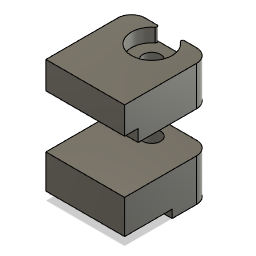
Korthållare_bak v4 (Autodesk Fusion 360 design; units mm, degrees)
Autodesk Fusion 360 part; units mm, degrees
sketch "Sketch1" plane through (0, 0, 0) normal (1, 0, 0) x (0, 0, -1)
  line L0 (0, 0) -> (-5.6, 0)
  line L1 (-5.6, 0) -> (-5.6, 1.2)
  line L2 (-5.6, 1.2) -> (-12.6, 1.2)
  line L3 (-12.6, 1.2) -> (-12.6, 6.2)
  line L4 (-12.6, 6.2) -> (0, 6.2)
  line L5 (0, 6.2) -> (0, 0)
  line L6 (-12.6, 8) -> (-10.6, 8)
  line L7 (-10.6, 8) -> (-10.6, 6.2)
  line L8 (-12.6, 8) -> (-12.6, 12)
  line L9 (-12.6, 12) -> (0, 12)
  line L10 (0, 12) -> (0, 6.2)
  dimension "d1" = 5.6
  dimension "d2" = 1.2
  dimension "d4" = 5
  dimension "d5" = 1.8
  dimension "d6" = 2
  dimension "d7" = 4
  dimension "d24" = 5
  constraint coincident L0.start L5.end
  constraint horizontal L0
  constraint perpendicular L0 L1
  constraint perpendicular L1 L2
  constraint perpendicular L2 L3
  constraint perpendicular L3 L4
  constraint vertical L5
  constraint horizontal L6
  constraint coincident L4 L7.end
  constraint perpendicular L4 L7
  constraint perpendicular L6 L8
  constraint perpendicular L8 L9
  constraint vertical L10
  constraint collinear L3 L8
  measures "d1" distance of L0.start L0.end
  measures "d2" distance of L0.end L1.end
  measures "d4" distance of L2.end L3.end
  measures "d5" distance of L6.end L7.end
  measures "d6" distance of L6.start L6.end
  measures "d7" distance of L6 L9
  measures "d24" distance of L1 L7
extrude "Extrude1" add sketch "Sketch1" along normal blind 11.6 contours L0 L1 L2 L3 L4 L5 makes body 1
extrude "Extrude2" add sketch "Sketch1" along normal blind 11.6 separate body contours L4 L6 L7 L8 L9 L10 makes body 2
sketch "Sketch2" plane through (0, 12, 0) normal (0, 1, 0) x (-1, 0, 0)
  line L0 (0, 0) -> (0, 12.6)
  line L1 (0, 12.6) -> (-11.6, 12.6)
  line L2 (-11.6, 12.6) -> (-11.6, 0)
  line L3 (-11.6, 0) -> (0, 0)
  circle A0 centre (-5.8, 2.8) radius 1.3
  line L4 (-5.8, 2.8) -> (-5.8, 0) construction
  circle A1 centre (-5.8, 2.8) radius 3
  dimension "d12" = 2.6
  dimension "d15" = 2.8
  dimension "d20" = 6
  constraint coincident A0.centre L4.start
  constraint midpoint L3 L4.end
  constraint perpendicular L3 L4
  constraint concentric A0 A1
  measures "d12" diameter of A0
  measures "d15" distance of A0.centre L4.end
  measures "d20" diameter of A1
extrude "Extrude3" cut sketch "Sketch2" against normal blind 18 contours A0 bodies 1 2
extrude "Extrude5" cut sketch "Sketch2" against normal blind 2 contours L3 A1 | L3 A1 bodies 2
sketch "Sketch3" plane through (0, 0, 0) normal (0, -1, 0) x (1, 0, 0)
  circle A0 centre (5.8, 2.8) radius 1.3
  line L0 (0, 5.6) -> (0, 0)
  line L1 (0, 0) -> (11.6, 0)
  line L2 (11.6, 0) -> (11.6, 5.6)
  line L3 (11.6, 5.6) -> (0, 5.6)
  line L4 (7.0124, 0.7) -> (8.2249, 2.8)
  line L5 (8.2249, 2.8) -> (7.0124, 4.9)
  line L6 (7.0124, 4.9) -> (4.5876, 4.9)
  line L7 (4.5876, 4.9) -> (3.3751, 2.8)
  line L8 (3.3751, 2.8) -> (4.5876, 0.7)
  line L9 (4.5876, 0.7) -> (7.0124, 0.7)
  point P0 (5.8, 2.8)
  dimension "d16" = 4.2
  constraint coincident P0 A0.centre
  constraint horizontal L9
  measures "d16" distance of L6 L9
extrude "Extrude4" cut sketch "Sketch3" against normal blind 4 contours L4 L5 L6 L7 L8 L9 bodies 1
move_body "Move1" bodies 1 to x (1, 0, 0) y (0, 1, 0) z (0, 0, 1) at (0, -6, 0)
fillet "Fillet2" radius 0.25 2 edges at (4.723, 11, 0) (6.877, 11, 0) on bodies 2
fillet "Fillet1" radius 2 4 edges at (11.6, -2.9, 0) (0, -2.9, 0) (0, 9.1, 0) (11.6, 9.1, 0) on bodies 1 2
named bodies: "Korthållare_bak_undre", "Korthållare_bak övre"
